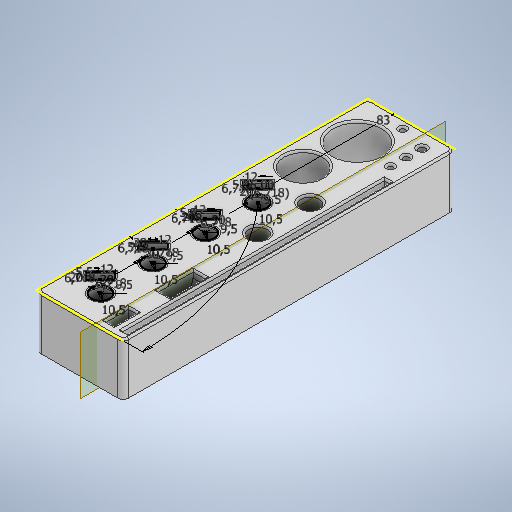
# Autodesk Inventor part: ToolBox
Saved by Autodesk Inventor 2025 (Build 290162000, 162)
## iProperties
Created: 2024-11-04
Part Number: ToolBox
Material: Типовые
Document SubType Name: Modeling
Designer: Makusimu
Density: 1 g/cm^3
Appearance: По умолчанию
Author: Makusimu
Autodesk Inventor part; units mm, degrees
ref_plane "YZ Plane" through (0, 0, 0) normal (1, 0, 0) x (0, 1, 0)
ref_plane "XZ Plane" through (0, 0, 0) normal (0, 1, 0) x (-1, 0, 0)
ref_plane "XY Plane" through (0, 0, 0) normal (0, 0, 1) x (1, 0, 0)
sketch "Эскиз1" plane through (0, 0, 0) normal (0, 1, 0) x (-1, 0, 0)
  line L0 (0, 0) -> (-50, 0)
  line L1 (-50, 0) -> (-50, -190)
  line L2 (-50, -190) -> (0, -190)
  line L3 (0, -190) -> (0, 0)
  dimension "d0" = 50
  dimension "d1" = 190
  constraints: 8 end point, 2 parallel, 1 horizontal, 1 perpendicular
  measures "d0" distance of L2.end L1.end
  measures "d1" distance of L1.end L0.end
extrude "Корпус" add sketch "Эскиз1" along normal blind 30
sketch "Эскиз2" plane through (0, 30, 0) normal (0, 1, 0) x (1, 0, 0)
  circle A0 centre (18, 166) radius 14
  line L0 (0, 190) -> (0, 0) projected
  line L1 (50, 190) -> (0, 190) projected
  dimension "d4" = 28
  dimension "d6" = 24
  dimension "d7" = 18
  constraints: 1 centre point
  measures "d4" diameter of A0
  measures "d6" distance from line of L1 A0.centre
  measures "d7" distance from line of L0 A0.centre
extrude "Клей" cut sketch "Эскиз2" against normal blind 29.1
sketch "Эскиз3" plane through (0, 30, 0) normal (0, 1, 0) x (1, 0, 0)
  circle A0 centre (15, 138) radius 10.95
  line L0 (0, 190) -> (0, 0) projected
  line L1 (50, 190) -> (0, 190) projected
  dimension "d10" = 21.9
  dimension "d12" = 52
  dimension "d13" = 15
  constraints: 1 centre point
  measures "d10" diameter of A0
  measures "d12" distance from line of L1 A0.centre
  measures "d13" distance from line of L0 A0.centre
extrude "Фаскосниматель" cut sketch "Эскиз3" against normal blind 29.1
sketch "Эскиз4" plane through (0, 30, 0) normal (0, 1, 0) x (1, 0, 0)
  circle A0 centre (25, 185) radius 1.5
  line L0 (0, 190) -> (0, 0) projected
  line L1 (50, 190) -> (0, 190) projected
  point P0 (25, 190)
  dimension "d16" = 3
  dimension "d17" = 25
  dimension "d18" = 5
  constraints: 1 centre point, 1 midpoint
  measures "d16" diameter of A0
  measures "d17" distance from line of L0 A0.centre
  measures "d18" distance of point (25, 190) A0.centre
extrude "Шомпол" cut sketch "Эскиз4" against normal blind 29.1
sketch "Эскиз5" plane through (0, 30, 0) normal (0, 1, 0) x (1, 0, 0)
  circle A0 centre (35, 122) radius 5.25
  line L0 (50, 0) -> (50, 190) projected
  line L1 (50, 190) -> (0, 190) projected
  point P0 (0, 0)
  dimension "d21" = 10.5
  dimension "d22" = 15
  dimension "d23" = 68
  constraints: 1 centre point
  measures "d21" diameter of A0
  measures "d22" distance from line of L0 A0.centre
  measures "d23" distance from line of L1 A0.centre
extrude "Лопатка" cut sketch "Эскиз5" against normal blind 30
sketch "Сопла" plane through (0, 30, 0) normal (0, 1, 0) x (1, 0, 0)
  circle A0 centre (20, 107) radius 5.25
  line L0 (0, 190) -> (0, 0) projected
  line L1 (5.1508, 113.364) -> (9.0398, 109.4749)
  line L2 (9.0398, 109.4749) -> (17.5251, 117.9602)
  line L3 (17.5251, 117.9602) -> (13.636, 121.8492)
  line L4 (13.636, 121.8492) -> (5.1508, 113.364)
  line L5 (0, 0) -> (50, 0) projected
  circle A1 centre (20, 77) radius 5.25
  line L6 (5.1508, 83.364) -> (9.0398, 79.4749)
  line L7 (9.0398, 79.4749) -> (17.5251, 87.9602)
  line L8 (17.5251, 87.9602) -> (13.636, 91.8492)
  line L9 (13.636, 91.8492) -> (5.1508, 83.364)
  circle A2 centre (20, 47) radius 5.25
  line L10 (5.1508, 53.364) -> (9.0398, 49.4749)
  line L11 (9.0398, 49.4749) -> (17.5251, 57.9602)
  line L12 (17.5251, 57.9602) -> (13.636, 61.8492)
  line L13 (13.636, 61.8492) -> (5.1508, 53.364)
  line L14 (17.5251, 27.9602) -> (13.636, 31.8492)
  line L15 (13.636, 31.8492) -> (5.1508, 23.364)
  line L16 (5.1508, 23.364) -> (9.0398, 19.4749)
  line L17 (9.0398, 19.4749) -> (17.5251, 27.9602)
  circle A3 centre (20, 17) radius 5.25
  line L18 (50, 190) -> (0, 190) projected
  point P0 (13.2825, 113.7175)
  point P1 (13.2825, 83.7175)
  point P2 (13.2825, 53.7175)
  point P3 (13.2825, 23.7175)
  dimension "d89" = 150
  dimension "d26" = 10.5
  dimension "d27" = 20
  dimension "d28" = 45
  dimension "d29" = 9.5
  dimension "d35" = 10.5
  dimension "d36" = 9.5
  dimension "d37" = 20
  dimension "d38" = 30
  dimension "d39" = 10.5
  dimension "d40" = 9.5
  dimension "d41" = 20
  dimension "d42" = 30
  dimension "d43" = 10.5
  dimension "d44" = 9.5
  dimension "d45" = 20
  dimension "d46" = 30
  dimension "d47" = 83
  dimension "d48" = 6.7175
  dimension "d49" = 6.7175
  dimension "d50" = 6.7175
  dimension "d51" = 6.7175
  dimension "d52" = 6.7175
  dimension "d53" = 6.7175
  dimension "d54" = 6.7175
  dimension "d55" = 6.7175
  dimension "d98" = 12
  dimension "d99" = 5.5
  dimension "d100" = 12
  dimension "d101" = 5.5
  dimension "d102" = 12
  dimension "d103" = 5.5
  dimension "d104" = 12
  dimension "d105" = 5.5
  constraints: 32 end point, 8 parallel, 4 centre point, 4 midpoint, 4 perpendicular
  measures "d26" diameter of A0
  measures "d27" distance from line of L0 A0.centre
  measures "d28" angle of L5 L2
  measures "d29" distance from line of A0.centre L2
  measures "d35" diameter of A1
  measures "d36" distance from line of A1.centre L7
  measures "d37" distance from line of L0 A1.centre
  measures "d38" distance of A1.centre A0.centre
  measures "d39" diameter of A2
  measures "d40" distance from line of A2.centre L11
  measures "d41" distance from line of L0 A2.centre
  measures "d42" distance of A2.centre A1.centre
  measures "d43" diameter of A3
  measures "d44" distance from line of A3.centre L17
  measures "d45" distance from line of L0 A3.centre
  measures "d46" distance of A3.centre A2.centre
  measures "d47" distance from line of L18 A0.centre
  measures "d48" horizontal distance of point (13.282, 113.718) A0.centre
  measures "d49" horizontal distance of A0.centre point (13.282, 113.718)
  measures "d50" horizontal distance of point (13.282, 83.718) A1.centre
  measures "d51" horizontal distance of point (13.282, 83.718) A1.centre
  measures "d52" horizontal distance of point (13.282, 53.718) A2.centre
  measures "d53" horizontal distance of point (13.282, 53.718) A2.centre
  measures "d54" horizontal distance of point (13.282, 23.718) A3.centre
  measures "d55" horizontal distance of point (13.282, 23.718) A3.centre
  measures "d98" distance of L3.end L1.start
  measures "d99" distance between parallel lines of L2 L4
  measures "d100" distance between parallel lines of L6 L8
  measures "d101" distance between parallel lines of L9 L7
  measures "d102" distance between parallel lines of L12 L10
  measures "d103" distance between parallel lines of L11 L13
  measures "d104" distance between parallel lines of L14 L16
  measures "d105" distance between parallel lines of L15 L17
extrude "Сопла - радиатор" cut sketch "Сопла" against normal blind 30 contours A0 | A1 | A2 | A3
extrude "Сопла - коннектор" cut sketch "Сопла" against normal blind 5.2 contours L4 L3 L2 L1 | L9 L8 L7 L6 | L13 L12 L11 L10 | L17 L16 L15 L14
sketch "Эскиз7" plane through (0, 30, 0) normal (0, 1, 0) x (1, 0, 0)
  line L0 (35, 18) -> (40, 18)
  line L1 (40, 18) -> (40, 5)
  line L2 (40, 5) -> (35, 5)
  line L3 (35, 5) -> (35, 18)
  line L4 (0, 0) -> (50, 0) projected
  line L5 (0, 190) -> (0, 0) projected
  point P0 (37.5, 5)
  point P1 (35, 11.5)
  dimension "d60" = 5
  dimension "d61" = 13
  dimension "d62" = 5
  dimension "d63" = 35
  constraints: 8 end point, 2 midpoint, 2 parallel, 1 horizontal, 1 perpendicular
  measures "d60" distance of L1.end L2.end
  measures "d61" distance of L0.end L1.end
  measures "d62" distance from line of L4 point (37.5, 5)
  measures "d63" distance from line of L5 point (35, 11.5)
extrude "Флешка" cut sketch "Эскиз7" against normal blind 12
sketch "Эскиз8" plane through (0, 30, 0) normal (0, 1, 0) x (1, 0, 0)
  circle A0 centre (35, 92) radius 5.25
  line L0 (50, 0) -> (50, 190) projected
  line L1 (50, 190) -> (0, 190) projected
  point P0 (0, 0)
  dimension "d66" = 10.5
  dimension "d67" = 15
  dimension "d68" = 98
  constraints: 1 centre point
  measures "d66" diameter of A0
  measures "d67" distance from line of L0 A0.centre
  measures "d68" distance from line of L1 A0.centre
extrude "Скальпель" cut sketch "Эскиз8" against normal blind 30
ref_plane "РабПлоскость2" through (35, 0, -190) normal (-1, 0, 0) x (0, 0, 1)
sketch "Эскиз11" plane through (35, 0, -190) normal (-1, 0, 0) x (0, 0, 1)
  line L0 (155, 30) -> (155, 26)
  line L1 (155, 26) -> (147, 0.9)
  line L2 (147, 0.9) -> (143, 0.9)
  line L3 (143, 0.9) -> (135, 26)
  line L4 (135, 26) -> (135, 30)
  line L5 (135, 30) -> (155, 30)
  line L6 (190, 30) -> (0, 30) projected
  line L7 (190, 0) -> (190, 30) projected
  point P0 (145, 30)
  point P1 (145, 0.9)
  dimension "d78" = 4
  dimension "d79" = 29.1
  dimension "d80" = 0
  dimension "d81" = 4
  dimension "d82" = 4
  dimension "d83" = 35
  dimension "d84" = 20
  dimension "d85" = 10
  constraints: 12 end point, 2 midpoint, 2 perpendicular, 1 parallel, 1 vertical
  measures "d78" distance of L1.end L2.end
  measures "d79" distance of point (145, 30) point (145, 0.9)
  measures "d80" distance between parallel lines of L6 L5
  measures "d81" distance of L0.start L0.end
  measures "d82" distance of L3.end L4.end
  measures "d83" distance from line of L7 L0.start
  measures "d84" distance between parallel lines of L0 L4
  measures "d85" distance from line of L0 point (145, 0.9)
extrude "Кусачки" cut sketch "Эскиз11" against normal blind 7
sketch "Эскиз12" plane through (0, 30, 0) normal (0, 1, 0) x (1, 0, 0)
  line L0 (44.5, 5) -> (47.5, 5)
  line L1 (47.5, 5) -> (47.5, 155)
  line L2 (47.5, 155) -> (44.5, 155)
  line L3 (44.5, 155) -> (44.5, 5)
  line L4 (50, 0) -> (50, 190) projected
  line L5 (0, 0) -> (50, 0) projected
  dimension "d88" = 3
  dimension "d89" = 150
  dimension "d90" = 2.5
  dimension "d91" = 5
  constraints: 8 end point, 2 parallel, 1 horizontal, 1 perpendicular
  measures "d88" distance of L2.end L1.end
  measures "d89" distance of L1.end L0.end
  measures "d90" distance between parallel lines of L4 L1
  measures "d91" distance from line of L0.start L5
extrude "Клипсы" cut sketch "Эскиз12" against normal blind 15
fillet "Сопряжение1" radius 1 38 edges at (7.0953, 30, -21.4194) (9.3934, 30, -27.6066) (15.5806, 30, -29.9047) (13.2825, 30, -23.7175) (7.0953, 30, -51.4194) (9.3934, 30, -57.6066) (15.5806, 30, -59.9047) (13.2825, 30, -53.7175) (7.0953, 30, -81.4194) (9.3934, 30, -87.6066) (15.5806, 30, -89.9047) (13.2825, 30, -83.7175) (7.0953, 30, -111.4194) (9.3934, 30, -117.6066) (15.5806, 30, -119.9047) (13.2825, 30, -113.7175) (14.75, 30, -17) (14.75, 30, -47) (14.75, 30, -77) (14.75, 30, -107) (4.05, 30, -138) (4.05, 0.9, -138) (4, 30, -166) (4, 0.9, -166) (29.75, 30, -92) (29.75, 30, -122) (35, 30, -11.5) (37.5, 30, -18) (40, 30, -11.5) (37.5, 30, -5) (44.5, 30, -80) (46, 30, -5) (47.5, 30, -80) (46, 30, -155) (35, 30, -45) (38.5, 30, -55) (42, 30, -45) (38.5, 30, -35)
fillet "Сопряжение2" radius 3 4 edges at (0, 15, -190) (50, 15, -190) (0, 15, 0) (50, 15, 0)
fillet "Сопряжение3" radius 1 8 edges at (49.1213, 30, -0.8787) (50, 30, -95) (49.1213, 30, -189.1213) (25, 30, -190) (0.8787, 30, -189.1213) (0, 30, -95) (0.8787, 30, -0.8787) (25, 30, 0)
fillet "Сопряжение4" radius 1 1 edges at (23.5, 30, -185)
sketch "Эскиз13" plane through (0, 30, 0) normal (0, 1, 0) x (1, 0, 0)
  circle A0 centre (40, 181) radius 2
  circle A1 centre (40, 172) radius 1.75
  circle A2 centre (40, 163) radius 1.5
  line L0 (47, 190) -> (3, 190) projected
  line L1 (49, 187) -> (49, 3) projected
  line L2 (50, 3) -> (50, 187) projected
  point P0 (0, 0)
  dimension "d107" = 4
  dimension "d108" = 9
  dimension "d109" = 9
  dimension "d110" = 9
  dimension "d112" = 10
  dimension "d113" = 10
  dimension "d114" = 10
  dimension "d115" = 3.5
  dimension "d116" = 3
  constraints: 3 centre point
  measures "d107" diameter of A0
  measures "d108" distance from line of L0 A0.centre
  measures "d109" distance of A0.centre A1.centre
  measures "d110" distance of A1.centre A2.centre
  measures "d112" distance from line of L2 A2.centre
  measures "d113" distance from line of L2 A1.centre
  measures "d114" distance from line of L2 A0.centre
  measures "d115" diameter of A1
  measures "d116" diameter of A2
extrude "Шестигранники" cut sketch "Эскиз13" against normal blind 30
fillet "Сопряжение5" radius 1 3 edges at (38, 30, -181) (38.25, 30, -172) (38.5, 30, -163)
